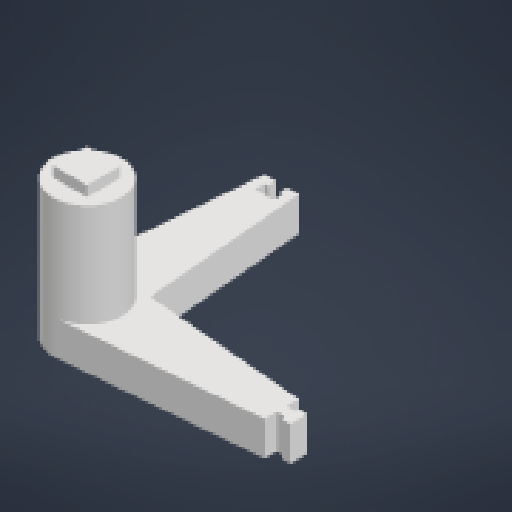
# Autodesk Inventor part: Leg_v1
Saved by Autodesk Inventor 2026 (Build 300175050, 175E)
## iProperties
Created: 2026-04-01
Part Number: Leg_v1
Material: Generic
Document SubType Name: Modeling
Designer: sniel
Density: 1 g/cm^3
Appearance: Default
Author: sniel
Autodesk Inventor part; units mm, degrees
ref_plane "YZ Plane" through (0, 0, 0) normal (1, 0, 0) x (0, 1, 0)
ref_plane "XZ Plane" through (0, 0, 0) normal (0, 1, 0) x (-1, 0, 0)
ref_plane "XY Plane" through (0, 0, 0) normal (0, 0, 1) x (1, 0, 0)
sketch "Sketch1" plane through (0, 0, 0) normal (0, 1, 0) x (-1, 0, 0)
  line L0 (4.9, 4.9) -> (-4.9, 4.9)
  line L1 (-4.9, 4.9) -> (-4.9, -4.9)
  line L2 (-4.9, -4.9) -> (4.9, -4.9)
  line L3 (4.9, -4.9) -> (4.9, 4.9)
  line L4 (4.9, 4.9) -> (-4.9, -4.9) construction
  line L5 (-4.9, 4.9) -> (4.9, -4.9) construction
  point P0 (0, 0)
  dimension "d0" = 9.8
  dimension "d1" = 9.8
  constraints: 12 end point, 2 midpoint, 2 parallel, 1 horizontal, 1 perpendicular
  measures "d0" distance of L2.end L1.end
  measures "d1" distance of L1.end L0.end
extrude "Extrusion1" add sketch "Sketch1" against normal blind 3
sketch "Sketch2" plane through (0, -3, 0) normal (0, -1, 0) x (1, 0, 0)
  circle A0 centre (0, 0) radius 10
  dimension "d4" = 20
  constraints: 1 centre point, 1 coincident
  measures "d4" diameter of A0
extrude "Extrusion2" add sketch "Sketch2" along normal blind 30
sketch "Sketch3" plane through (0, -33, 0) normal (0, -1, 0) x (1, 0, 0)
  arc A0 (56.6685, -50.6545) -> (56.6685, -62.6825) centre (56.6685, -56.6685) ccw projected
  line L0 (56.6685, -56.6685) -> (0, -56.6685)
  line L1 (0, -56.6685) -> (0, 0)
  circle A1 centre (0, 0) radius 10
  circle A2 centre (0, 0) radius 10 projected
  line L2 (0, -56.6685) -> (-5, -56.6685)
  line L3 (-5, -56.6685) -> (-9.9607, -0.8858)
  line L4 (56.6685, 5) -> (0.8858, 9.9607)
  line L5 (0, -56.6685) -> (5, -56.6685)
  line L6 (56.6685, -5) -> (0.8858, -9.9607)
  line L7 (5, -56.6685) -> (9.9607, -0.8858)
  line L8 (56.6685, 5) -> (112.4513, 9.9607)
  line L9 (56.6685, -5) -> (112.4513, -9.9607)
  line L10 (-5, -56.6685) -> (-9.9607, -112.4513)
  line L11 (5, -56.6685) -> (9.9607, -112.4513)
  line L12 (56.6685, 5) -> (56.6685, -5)
  line L13 (56.6685, 0) -> (56.6685, 1.5)
  line L14 (56.6685, 1.5) -> (59.1685, 1.5)
  line L15 (59.1685, 1.5) -> (59.1685, 2.5)
  line L16 (56.6685, 0) -> (56.6685, -1.5)
  line L17 (56.6685, -1.5) -> (59.1685, -1.5)
  line L18 (59.1685, -1.5) -> (59.1685, -2.5)
  line L19 (59.1685, -2.5) -> (61.6685, -2.5)
  line L20 (61.6685, -2.5) -> (61.6685, 2.5)
  line L21 (61.6685, 2.5) -> (59.1685, 2.5)
  line L22 (-1.5, -56.6685) -> (-1.5, -54.1685)
  line L23 (-1.5, -54.1685) -> (-2.5, -54.1685)
  line L24 (1.5, -56.6685) -> (1.5, -54.1685)
  line L25 (1.5, -54.1685) -> (2.5, -54.1685)
  line L26 (2.5, -54.1685) -> (2.5, -51.6685)
  line L27 (2.5, -51.6685) -> (-2.5, -51.6685)
  line L28 (-2.5, -51.6685) -> (-2.5, -54.1685)
  line L29 (-1.5, -56.6685) -> (1.5, -56.6685)
  line L30 (1.5, -56.6685) -> (1.65, -56.6685)
  line L31 (1.65, -56.6685) -> (1.65, -56.5185)
  line L32 (1.65, -56.5185) -> (1.5, -56.5185)
  line L33 (1.5, -56.5185) -> (1.5, -56.6685)
  line L34 (1.5, -54.1685) -> (1.65, -54.1685)
  line L35 (1.65, -54.1685) -> (1.65, -54.3185)
  line L36 (1.65, -54.3185) -> (1.5, -54.3185)
  line L37 (1.5, -54.3185) -> (1.5, -54.1685)
  line L38 (2.5, -54.1685) -> (2.65, -54.1685)
  line L39 (2.65, -54.1685) -> (2.65, -54.3185)
  line L40 (2.65, -54.3185) -> (2.5, -54.3185)
  line L41 (2.5, -54.3185) -> (2.5, -54.1685)
  line L42 (2.5, -51.6685) -> (2.65, -51.6685)
  line L43 (2.65, -51.6685) -> (2.65, -51.5185)
  line L44 (2.65, -51.5185) -> (2.5, -51.5185)
  line L45 (2.5, -51.5185) -> (2.5, -51.6685)
  line L46 (-2.5, -51.6685) -> (-2.65, -51.6685)
  line L47 (-2.65, -51.6685) -> (-2.65, -51.5185)
  line L48 (-2.65, -51.5185) -> (-2.5, -51.5185)
  line L49 (-2.5, -51.5185) -> (-2.5, -51.6685)
  line L50 (-2.5, -54.1685) -> (-2.65, -54.1685)
  line L51 (-2.65, -54.1685) -> (-2.65, -54.3185)
  line L52 (-2.65, -54.3185) -> (-2.5, -54.3185)
  line L53 (-2.5, -54.3185) -> (-2.5, -54.1685)
  line L54 (-1.5, -54.1685) -> (-1.65, -54.1685)
  line L55 (-1.65, -54.1685) -> (-1.65, -54.3185)
  line L56 (-1.65, -54.3185) -> (-1.5, -54.3185)
  line L57 (-1.5, -54.3185) -> (-1.5, -54.1685)
  line L58 (-1.5, -56.6685) -> (-1.65, -56.6685)
  line L59 (-1.65, -56.6685) -> (-1.65, -56.5185)
  line L60 (-1.65, -56.5185) -> (-1.5, -56.5185)
  line L61 (-1.5, -56.5185) -> (-1.5, -56.6685)
  line L62 (2.65, -51.6685) -> (2.65, -54.1685)
  line L63 (2.5, -51.5185) -> (-2.5, -51.5185)
  line L64 (-2.65, -51.6685) -> (-2.65, -54.1685)
  line L65 (-1.65, -54.3185) -> (-2.5, -54.3185)
  line L66 (-1.65, -54.3185) -> (-1.65, -56.5185)
  line L67 (1.65, -54.3185) -> (2.5, -54.3185)
  line L68 (1.65, -54.3185) -> (1.65, -56.5185)
  point P0 (0.8858, 9.9607)
  point P1 (0.8858, -9.9607)
  point P2 (0, -56.6685)
  point P3 (9.2196, -9.2196)
  point P4 (-9.9607, -0.8858)
  dimension "d8" = 5
  dimension "d23" = 1.5
  dimension "d24" = 2.5
  dimension "d25" = 1
  dimension "d26" = 1.5
  dimension "d27" = 2.5
  dimension "d28" = 1
  dimension "d29" = 2.5
  dimension "d32" = 2.5
  dimension "d33" = 1
  dimension "d34" = 2.5
  dimension "d35" = 1
  dimension "d36" = 2.5
  dimension "d37" = 0.15
  dimension "d38" = 0.15
  dimension "d39" = 0.15
  dimension "d40" = 0.15
  dimension "d41" = 0.15
  dimension "d42" = 0.15
  dimension "d43" = 0.15
  dimension "d44" = 0.15
  dimension "d45" = 0.15
  dimension "d46" = 0.15
  dimension "d47" = 0.15
  dimension "d48" = 0.15
  dimension "d49" = 0.15
  dimension "d50" = 0.15
  dimension "d51" = 0.15
  dimension "d52" = 0.15
  constraints: 138 end point, 23 perpendicular, 16 parallel, 9 horizontal, 4 point on circle, 4 tangent, 3 point on line, 2 midpoint, 2 symmetric about line, 2 vertical, 1 centre point, 1 coincident
  measures "d8" distance of L0.end L5.end
  measures "d23" distance of L13.start L13.end
  measures "d24" distance of L13.end L14.end
  measures "d25" distance of L14.end L15.end
  measures "d26" distance of L13.start L16.end
  measures "d27" distance of L16.end L17.end
  measures "d28" distance of L17.end L18.end
  measures "d29" distance of L18.end L19.end
  measures "d32" distance of L22.start L22.end
  measures "d33" distance of L22.end L23.end
  measures "d34" distance of L24.start L24.end
  measures "d35" distance of L24.end L25.end
  measures "d36" distance of L25.end L27.start
  measures "d37" distance of L32.end L31.end
  measures "d38" distance of L31.end L30.end
  measures "d39" distance of L35.end L36.end
  measures "d40" distance of L34.end L35.end
  measures "d41" distance of L39.end L40.end
  measures "d42" distance of L38.end L39.end
  measures "d43" distance of L44.end L43.end
  measures "d44" distance of L43.end L42.end
  measures "d45" distance of L47.end L48.end
  measures "d46" distance of L46.end L47.end
  measures "d47" distance of L52.end L51.end
  measures "d48" distance of L51.end L50.end
  measures "d49" distance of L56.end L55.end
  measures "d50" distance of L55.end L54.end
  measures "d51" distance of L59.end L60.end
  measures "d52" distance of L58.end L59.end
extrude "Extrusion3" add sketch "Sketch3" along normal blind 10 contours L0 L31 L68 L67 L40 L39 L62 L43 L44 L63 L1 A1 L6 L7 | L7 A1 L4 L12 L6 | L6 A1 L7 | A1 | L12 L14 L15 L21 L20 L19 L18 L17 | L1 L63 L48 L47 L64 L51 L52 L65 L66 L59 L2 L3 A1
body "Solid1"
